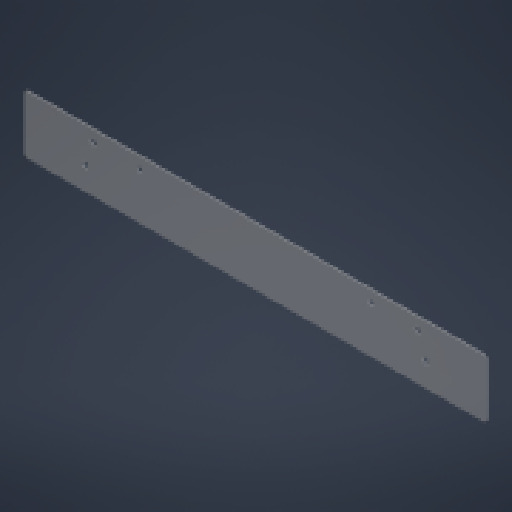
# Autodesk Inventor part: wedge
Saved by Autodesk Inventor 2024 (Build 280153000, 153)
## iProperties
Created: 2023-11-18
Part Number: wedge
Material: Polycarbonate, Clear
Document SubType Name: Modeling
Designer: macbook
Density: 1.2 g/cm^3
Appearance: Polycarbonate - Clear(1)
Author: macbook
Autodesk Inventor part; units mm, degrees
ref_plane "YZ Plane" through (0, 0, 0) normal (1, 0, 0) x (0, 1, 0)
ref_plane "XZ Plane" through (0, 0, 0) normal (0, 1, 0) x (-1, 0, 0)
ref_plane "XY Plane" through (0, 0, 0) normal (0, 0, 1) x (1, 0, 0)
sketch "Sketch1" plane through (0, 0, 0) normal (0, 0, 1) x (1, 0, 0)
  line L0 (-381, -3.175) -> (-381, 38.1)
  line L1 (-377.825, 50.8) -> (-3.175, 50.8)
  line L2 (0, 38.1) -> (0, 0)
  line L3 (-381, 0) -> (-381, -6.35)
  line L4 (-377.825, -6.35) -> (-3.175, -6.35)
  line L5 (0, -3.175) -> (0, 0)
  arc A0 (-381, -3.175) -> (-377.825, -6.35) centre (-377.825, -3.175) ccw
  arc A1 (-377.825, 50.8) -> (-381, 47.625) centre (-377.825, 47.625) ccw
  arc A2 (0, 47.625) -> (-3.175, 50.8) centre (-3.175, 47.625) ccw
  arc A3 (-3.175, -6.35) -> (0, -3.175) centre (-3.175, -3.175) ccw
  line L6 (-381, 50.8) -> (-381, 41.275)
  line L7 (-377.825, 41.275) -> (-3.175, 41.275)
  arc A4 (-377.825, 41.275) -> (-381, 38.1) centre (-377.825, 38.1) ccw
  arc A5 (0, 38.1) -> (-3.175, 41.275) centre (-3.175, 38.1) ccw
  point P0 (0, 50.8)
  point P1 (0, -6.35)
  point P2 (0, 41.275)
  dimension "d1" = 50.8
  dimension "d7" = 6.35
  dimension "d19" = 3.175
  dimension "d20" = 3.175
  dimension "d25" = 9.525
  dimension "d26" = 3.175
  constraints: 16 end point, 14 point on line, 12 point on circle, 12 tangent, 6 centre point, 4 perpendicular, 3 equal radius, 2 vertical, 1 horizontal
  measures "d1" distance of L3.start L6.start
  measures "d7" distance of L3.start L3.end
  measures "d19" radius of A0
  measures "d20" radius of A3
  measures "d25" distance of L6.start L6.end
  measures "d26" radius of A4
extrude "Extrusion1" add sketch "Sketch1" along normal blind 1.5875
sketch "Sketch2" plane through (0, 0, 1.5875) normal (0, 0, 1) x (1, 0, 0)
  line L0 (-381, 50.8) -> (-323.85, 50.8)
  line L1 (-323.85, 50.8) -> (-273.05, 50.8)
  line L2 (-381, 0) -> (-330.2, 0)
  line L3 (-323.85, 50.8) -> (-323.85, 31.75)
  line L4 (-190.5, 50.8) -> (-190.5, -6.35)
  line L5 (0, 50.8) -> (-57.15, 50.8)
  line L6 (-57.15, 50.8) -> (-107.95, 50.8)
  line L7 (0, 0) -> (-50.8, 0)
  line L8 (-57.15, 50.8) -> (-57.15, 31.75)
  line L9 (-273.05, 50.8) -> (-285.75, 50.8)
  line L10 (-3.175, 50.8) -> (-377.825, 50.8) projected
  line L11 (-285.75, 50.8) -> (-285.75, 31.75)
  line L12 (-107.95, 50.8) -> (-95.25, 50.8)
  line L13 (-95.25, 50.8) -> (-95.25, 31.75)
  line L14 (-50.8, 0) -> (-50.8, 12.7)
  line L15 (-330.2, 0) -> (-330.2, 12.7)
  line L16 (0, 50.8) -> (0, 41.275)
  line L17 (0, -3.175) -> (0, 47.625) projected
  line L18 (-381, 38.1) -> (-381, -3.175) projected
  line L19 (-381, 41.275) -> (0, 41.275)
  point P0 (-381, 47.625)
  dimension "d4" = 57.15
  dimension "d5" = 50.8
  dimension "d11" = 50.8
  dimension "d21" = 12.7
  dimension "d22" = 12.7
  dimension "d23" = 12.7
  dimension "d24" = 9.525
  constraints: 34 end point, 7 symmetric about line, 6 coincident, 3 perpendicular, 3 vertical, 2 point on line, 1 horizontal, 3 other
  measures "d4" distance of L0.start L0.end
  measures "d5" distance of L0.end L1.end
  measures "d11" distance of L2.start L2.end
  measures "d21" distance of L1.end L9.end
  measures "d22" distance of L6.end L12.end
  measures "d23" distance of L7.end L14.end
  measures "d24" distance of L5.start L16.end
hole "Hole1" at (-323.85, 31.75, 1.5875) at (-57.15, 31.75, 1.5875) at (-285.75, 31.75, 1.5875) at (-95.25, 31.75, 1.5875) at (-330.2, 12.7, 1.5875) at (-50.8, 12.7, 1.5875) direction (0, 0, -1) diameter 4.7625 end through all
body "Solid1"
